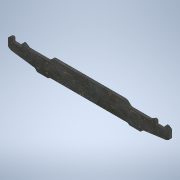
# Autodesk Inventor part: MK3 Rear Plate
Saved by Autodesk Inventor 2023 (Build 270158000, 158)
## iProperties
Created: 2019-05-27
Part Number: MK3 Rear Plate
Material: Steel
Document SubType Name: Modeling
Designer: Parker
Density: 7.85 g/cm^3
Appearance: Plate
Author: Parker
Revision Number: ANY
Autodesk Inventor part; units mm, degrees
ref_plane "YZ Plane" through (0, 0, 0) normal (1, 0, 0) x (0, 1, 0)
ref_plane "XZ Plane" through (0, 0, 0) normal (0, 1, 0) x (-1, 0, 0)
ref_plane "XY Plane" through (0, 0, 0) normal (0, 0, 1) x (1, 0, 0)
sketch "Sketch5" plane through (0, 0, 0) normal (0, 0, 1) x (1, 0, 0)
  line L0 (-212.5, -25) -> (212.5, -25)
  line L1 (212.5, -25) -> (212.5, 25)
  line L2 (212.5, 25) -> (-212.5, 25)
  line L3 (-212.5, 25) -> (-212.5, -25)
  line L4 (-212.5, -25) -> (212.5, 25) construction
  line L5 (212.5, -25) -> (-212.5, 25) construction
  point P0 (0, 0)
  dimension "d22" = 425
  dimension "d23" = 50
  constraints: 12 end point, 2 midpoint, 2 parallel, 1 horizontal, 1 perpendicular
  measures "d22" distance of L1.end L2.end
  measures "d23" distance of L2.end L0.start
extrude "Extrusion3" add sketch "Sketch5" along normal blind 6.35
sketch "Sketch6" plane through (0, 0, 0) normal (0, 0, -1) x (-1, 0, 0)
  circle A0 centre (74, 14.9487) radius 2.75
  circle A1 centre (85, 10.04) radius 2.75
  circle A2 centre (96, 14.9487) radius 2.75
  circle A3 centre (-74, 14.9487) radius 2.75
  circle A4 centre (-85, 10.04) radius 2.75
  circle A5 centre (-96, 14.9487) radius 2.75
  circle A6 centre (-19.65, 8.0332) radius 2.75
  circle A7 centre (2.35, 8.037) radius 2.75
  circle A8 centre (2.35, -13.963) radius 2.75
  circle A9 centre (-19.6575, -13.9668) radius 2.75
  point P0 (-19.6575, -16.9668)
  point P1 (-19.65, 5.0332)
  point P2 (2.35, 5.037)
  point P3 (2.35, -16.963)
  constraints: 10 centre point, 20 other
hole "Hole2" at (96, 14.9487, 0) at (85, 10.04, 0) at (74, 14.9487, 0) at (-74, 14.9487, 0) at (-85, 10.04, 0) at (-96, 14.9487, 0) at (-2.35, -13.963, 0) at (19.6575, -13.9668, 0) at (19.65, 8.0332, 0) at (-2.35, 8.037, 0) direction (0, 0, 1) diameter 3.2 end through all
sketch "Sketch7" plane through (0, 0, 0) normal (0, 0, -1) x (-1, 0, 0)
  circle A0 centre (-133.6, 8.1) radius 3.825
  circle A1 centre (-110.4, 8.1) radius 3.825
  circle A2 centre (-110.4, -15.1) radius 3.825
  circle A3 centre (-133.6, -15.1) radius 3.825
  circle A4 centre (133.6, -15.1) radius 3.825
  circle A5 centre (110.4, -15.1) radius 3.825
  circle A6 centre (110.4, 8.1) radius 3.825
  circle A7 centre (133.6, 8.1) radius 3.825
  point P0 (0, 0)
  constraints: 8 centre point, 16 other
hole "Hole3" at (133.6, 8.1, 0) at (133.6, -15.1, 0) at (110.4, -15.1, 0) at (110.4, 8.1, 0) at (-110.4, 8.1, 0) at (-133.6, 8.1, 0) at (-133.6, -15.1, 0) at (-110.4, -15.1, 0) direction (0, 0, 1) diameter 5.4 end through all
sketch "Sketch8" plane through (0, 0, 0) normal (0, 0, -1) x (-1, 0, 0)
  circle A0 centre (-208.5036, 13.3515) radius 1.7
  circle A1 centre (-208.5036, -3.1485) radius 1.7
  circle A2 centre (-167.5036, -3.1485) radius 1.7
  circle A3 centre (-167.5036, 13.3515) radius 1.7
  circle A4 centre (167.4964, 13.3515) radius 1.7
  circle A5 centre (167.4964, -3.1485) radius 1.7
  circle A6 centre (208.4964, -3.1485) radius 1.7
  circle A7 centre (208.4964, 13.3515) radius 1.7
  point P0 (0, 0)
  constraints: 8 centre point, 16 other
hole "Hole4" at (208.5036, 13.3515, 0) at (208.5036, -3.1485, 0) at (167.5036, -3.1485, 0) at (167.5036, 13.3515, 0) at (-167.4964, 13.3515, 0) at (-167.4964, -3.1485, 0) at (-208.4964, -3.1485, 0) at (-208.4964, 13.3515, 0) direction (0, 0, 1) diameter 2.2 end through all
sketch "Sketch9" plane through (0, 0, 0) normal (0, 0, -1) x (-1, 0, 0)
  arc A0 (-210.5036, 16.8156) -> (-210.5036, 9.8874) centre (-208.5036, 13.3515) ccw
  line L0 (-210.5036, 16.8156) -> (-205.1272, 20.2721)
  arc A1 (-204.9977, 20.3312) -> (-205.1272, 20.2721) centre (-204.8568, 19.8515) ccw
  arc A2 (-204.8568, 20.3515) -> (-204.9977, 20.3312) centre (-204.8568, 19.8515) ccw
  line L1 (-204.8568, 20.3515) -> (-202.0036, 20.3515)
  circle A3 centre (208.4964, -3.1485) radius 1.1 projected
  circle A4 centre (167.4964, 13.3515) radius 1.1 projected
  circle A5 centre (-167.5036, -3.1485) radius 1.1 projected
  circle A6 centre (-208.5036, 13.3515) radius 1.1 projected
  circle A7 centre (-208.5036, -3.1485) radius 1.1 projected
  circle A8 centre (-167.5036, 13.3515) radius 1.1 projected
  circle A9 centre (167.4964, -3.1485) radius 1.1 projected
  circle A10 centre (208.4964, 13.3515) radius 1.1 projected
  circle A11 centre (133.6, -15.1) radius 2.7 projected
  circle A12 centre (110.4, 8.1) radius 2.7 projected
  circle A13 centre (-110.4, -15.1) radius 2.7 projected
  circle A14 centre (-133.6, 8.1) radius 2.7 projected
  circle A15 centre (-133.6, -15.1) radius 2.7 projected
  circle A16 centre (-110.4, 8.1) radius 2.7 projected
  circle A17 centre (133.6, 8.1) radius 2.7 projected
  circle A18 centre (110.4, -15.1) radius 2.7 projected
  circle A19 centre (85, 10.04) radius 1.6 projected
  circle A20 centre (-74, 14.9487) radius 1.6 projected
  circle A21 centre (-96, 14.9487) radius 1.6 projected
  circle A22 centre (-85, 10.04) radius 1.6 projected
  circle A23 centre (74, 14.9487) radius 1.6 projected
  circle A24 centre (96, 14.9487) radius 1.6 projected
  line L2 (-212.5, -25) -> (-212.5, 25) projected
  line L3 (212.5, -25) -> (-212.5, -25) projected
  line L4 (212.5, 25) -> (212.5, -25) projected
  line L5 (-212.5, 25) -> (212.5, 25) projected
  line L6 (-174.0036, 20.3515) -> (-171.1505, 20.3515)
  arc A25 (-174.0036, 20.3515) -> (-174.448, 20.3015) centre (-174.0036, 18.3515) ccw
  arc A26 (-174.448, 20.3015) -> (-175.9536, 18.7959) centre (-174.0036, 18.3515) ccw
  arc A27 (-175.9536, 18.7959) -> (-176.0036, 18.3515) centre (-174.0036, 18.3515) ccw
  line L7 (-176.0036, 12.3515) -> (-176.0036, 18.3515)
  arc A28 (-201.5592, 20.3015) -> (-202.0036, 20.3515) centre (-202.0036, 18.3515) ccw
  arc A29 (-200.0536, 18.7959) -> (-201.5592, 20.3015) centre (-202.0036, 18.3515) ccw
  arc A30 (-200.0036, 18.3515) -> (-200.0536, 18.7959) centre (-202.0036, 18.3515) ccw
  line L8 (-200.0036, 18.3515) -> (-200.0036, 12.3515)
  line L9 (-198.0036, 10.3515) -> (-178.0036, 10.3515)
  circle A31 centre (-133.6, 8.1) radius 4.25
  circle A32 centre (-110.4, 8.1) radius 4.25
  line L10 (-161.2796, 14.1) -> (-106.2796, 14.1)
  line L11 (-106.2796, 14.1) -> (-95.3796, 25)
  arc A33 (-171.0096, 20.3312) -> (-171.1505, 20.3515) centre (-171.1505, 19.8515) ccw
  arc A34 (-170.8801, 20.2721) -> (-171.0096, 20.3312) centre (-171.1505, 19.8515) ccw
  line L12 (-170.8801, 20.2721) -> (-165.5036, 16.8156)
  line L13 (-165.5036, 16.8156) -> (-161.2796, 14.1)
  line L14 (-178.0036, 10.3515) -> (-178.0036, 10.3515)
  line L15 (-176.0036, 12.3515) -> (-176.0036, 12.3515)
  arc A35 (-178.0036, 10.3515) -> (-176.0036, 12.3515) centre (-178.0036, 12.3515) ccw
  line L16 (-198.0036, 10.3515) -> (-198.0036, 10.3515)
  line L17 (-200.0036, 12.3515) -> (-200.0036, 12.3515)
  arc A36 (-200.0036, 12.3515) -> (-198.0036, 10.3515) centre (-198.0036, 12.3515) ccw
  point P0 (0, 0)
  point P1 (-212.5, 13.5221)
  dimension "d47" = 6
  dimension "d48" = 45
  dimension "d49" = 2
  dimension "d50" = 2
  dimension "d51" = 55
  constraints: 29 end point, 26 point on circle, 15 centre point, 6 horizontal, 4 tangent, 2 perpendicular, 2 vertical, 1 collinear, 1 point on line, 49 other
  measures "d47" distance from line of L10 A31.centre
  measures "d48" angle of L5 L11
  measures "d49" radius of A35
  measures "d50" radius of A36
  measures "d51" distance of L10.start L10.end
extrude "Extrusion4" cut sketch "Sketch9" against normal through all contours A0 L2 L5 L11 L10 L13 L12 A34 A33 L6 A25 A26 A27 L7 A35 L9 A36 L8 A30 A29 A28 L1 A2 A1 L0
mirror "Mirror3" about plane through (0, 0, 0) normal (1, 0, 0) of "Extrusion4"
sketch "Sketch10" plane through (0, 0, 0) normal (0, 0, -1) x (-1, 0, 0)
  line L0 (212.5, -25) -> (-212.5, -25) projected
  line L1 (-136.6, -25) -> (-139.6, -19)
  line L2 (-139.6, -19) -> (-205.1276, -10.0894)
  line L3 (106.2796, 14.1) -> (95.3796, 25) projected
  line L4 (-95.3796, 25) -> (95.3796, 25) projected
  line L5 (-95.3796, 25) -> (-106.2796, 14.1) projected
  line L6 (-106.2796, 14.1) -> (-161.2796, 14.1) projected
  line L7 (-161.2796, 14.1) -> (-170.8801, 20.2721) projected
  arc A0 (-170.8801, 20.2721) -> (-171.1505, 20.3515) centre (-171.1505, 19.8515) ccw projected
  line L8 (-171.1505, 20.3515) -> (-174.0036, 20.3515) projected
  arc A1 (-174.0036, 20.3515) -> (-176.0036, 18.3515) centre (-174.0036, 18.3515) ccw projected
  line L9 (-176.0036, 18.3515) -> (-176.0036, 12.3515) projected
  arc A2 (-178.0036, 10.3515) -> (-176.0036, 12.3515) centre (-178.0036, 12.3515) ccw projected
  line L10 (-178.0036, 10.3515) -> (-198.0036, 10.3515) projected
  arc A3 (-200.0036, 12.3515) -> (-198.0036, 10.3515) centre (-198.0036, 12.3515) ccw projected
  line L11 (-200.0036, 12.3515) -> (-200.0036, 18.3515) projected
  arc A4 (-200.0036, 18.3515) -> (-202.0036, 20.3515) centre (-202.0036, 18.3515) ccw projected
  line L12 (-202.0036, 20.3515) -> (-204.8568, 20.3515) projected
  arc A5 (-204.8568, 20.3515) -> (-205.1272, 20.2721) centre (-204.8568, 19.8515) ccw projected
  line L13 (-205.1272, 20.2721) -> (-210.5036, 16.8156) projected
  arc A6 (-210.5036, 16.8156) -> (-212.5, 13.5221) centre (-208.5036, 13.3515) ccw projected
  line L14 (-212.5, -25) -> (-212.5, 13.5221) projected
  line L15 (212.5, -25) -> (-212.5, -25) projected
  line L16 (212.5, 13.5221) -> (212.5, -25) projected
  arc A7 (212.5, 13.5221) -> (210.5036, 16.8156) centre (208.5036, 13.3515) ccw projected
  line L17 (210.5036, 16.8156) -> (205.1272, 20.2721) projected
  arc A8 (205.1272, 20.2721) -> (204.8568, 20.3515) centre (204.8568, 19.8515) ccw projected
  line L18 (204.8568, 20.3515) -> (202.0036, 20.3515) projected
  arc A9 (202.0036, 20.3515) -> (200.0036, 18.3515) centre (202.0036, 18.3515) ccw projected
  line L19 (200.0036, 18.3515) -> (200.0036, 12.3515) projected
  arc A10 (198.0036, 10.3515) -> (200.0036, 12.3515) centre (198.0036, 12.3515) ccw projected
  line L20 (198.0036, 10.3515) -> (178.0036, 10.3515) projected
  arc A11 (176.0036, 12.3515) -> (178.0036, 10.3515) centre (178.0036, 12.3515) ccw projected
  line L21 (176.0036, 12.3515) -> (176.0036, 18.3515) projected
  arc A12 (176.0036, 18.3515) -> (174.0036, 20.3515) centre (174.0036, 18.3515) ccw projected
  line L22 (174.0036, 20.3515) -> (171.1505, 20.3515) projected
  arc A13 (171.1505, 20.3515) -> (170.8801, 20.2721) centre (171.1505, 19.8515) ccw projected
  line L23 (170.8801, 20.2721) -> (161.2796, 14.1) projected
  line L24 (161.2796, 14.1) -> (106.2796, 14.1) projected
  circle A14 centre (208.4964, -3.1485) radius 1.1 projected
  circle A15 centre (167.4964, 13.3515) radius 1.1 projected
  circle A16 centre (-167.5036, -3.1485) radius 1.1 projected
  circle A17 centre (-208.5036, 13.3515) radius 1.1 projected
  circle A18 centre (-208.5036, -3.1485) radius 1.1 projected
  circle A19 centre (-167.5036, 13.3515) radius 1.1 projected
  circle A20 centre (167.4964, -3.1485) radius 1.1 projected
  circle A21 centre (208.4964, 13.3515) radius 1.1 projected
  circle A22 centre (133.6, -15.1) radius 2.7 projected
  circle A23 centre (110.4, 8.1) radius 2.7 projected
  circle A24 centre (-110.4, -15.1) radius 2.7 projected
  circle A25 centre (-133.6, 8.1) radius 2.7 projected
  circle A26 centre (-133.6, -15.1) radius 2.7 projected
  circle A27 centre (-110.4, 8.1) radius 2.7 projected
  circle A28 centre (133.6, 8.1) radius 2.7 projected
  circle A29 centre (110.4, -15.1) radius 2.7 projected
  circle A30 centre (85, 10.04) radius 1.6 projected
  circle A31 centre (-74, 14.9487) radius 1.6 projected
  circle A32 centre (-96, 14.9487) radius 1.6 projected
  circle A33 centre (-85, 10.04) radius 1.6 projected
  circle A34 centre (74, 14.9487) radius 1.6 projected
  circle A35 centre (96, 14.9487) radius 1.6 projected
  arc A36 (-210.5036, 0.3156) -> (-210.5036, -6.6126) centre (-208.5036, -3.1485) ccw
  line L25 (-205.1276, -10.0894) -> (-210.5036, -6.6126)
  point P0 (0, 0)
  point P1 (-212.5, -3.3191)
  point P2 (-212.5, -25)
  dimension "d54" = 6
  dimension "d55" = 3
  dimension "d56" = 6
  constraints: 6 end point, 2 point on circle, 2 point on line, 1 centre point, 6 other
  measures "d54" horizontal distance of A26.centre L1.end
  measures "d55" horizontal distance of L1.end L1.start
  measures "d56" vertical distance of L1.start L1.end
extrude "Extrusion5" cut sketch "Sketch10" against normal blind 10 contours L0 L14 A36 L25 L2 L1
mirror "Mirror4" about plane through (0, 0, 0) normal (1, 0, 0) of "Extrusion5"
fillet "Fillet2" radius 10 2 edges at (205.1276, -10.0894, 3.175) (-205.1276, -10.0894, 3.175)
fillet "Fillet3" radius 10 2 edges at (-139.6, -19, 3.175) (139.6, -19, 3.175)
fillet "Fillet4" radius 10 6 edges at (106.2796, 14.1, 3.175) (95.3796, 25, 3.175) (-95.3796, 25, 3.175) (-106.2796, 14.1, 3.175) (-161.2796, 14.1, 3.175) (161.2796, 14.1, 3.175)
sketch "Sketch11" plane through (0, 0, 0) normal (0, 0, -1) x (-1, 0, 0)
  line L0 (136.6, -25) -> (-136.6, -25) projected
  line L1 (-106.9, -25) -> (-103.4, -21.5)
  line L2 (-103.4, -21.5) -> (103.4, -21.5)
  line L3 (103.4, -21.5) -> (106.9, -25)
  circle A0 centre (-110.4, -15.1) radius 2.7 projected
  circle A1 centre (110.4, -15.1) radius 2.7 projected
  point P0 (0, 0)
  dimension "d62" = 3.5
  dimension "d63" = 45
  dimension "d64" = 7
  dimension "d65" = 7
  constraints: 6 end point, 2 point on line, 1 parallel, 1 perpendicular
  measures "d62" distance between parallel lines of L0 L2
  measures "d63" angle of L0 L1
  measures "d64" horizontal distance of A0.centre L1.end
  measures "d65" horizontal distance of A1.centre L2.end
extrude "Extrusion6" cut sketch "Sketch11" against normal blind 10 contours L0 L1 L2 L3
fillet "Fillet5" radius 10 2 edges at (103.4, -21.5, 3.175) (-103.4, -21.5, 3.175)
sketch "Sketch12" plane through (0, 0, 0) normal (0, 0, -1) x (-1, 0, 0)
  circle A0 centre (110.4, -15.1) radius 2.7 projected
  line L0 (-99.2579, -21.5) -> (99.2579, -21.5) projected
  point P0 (0, 0)
  point P1 (80.4, -17.5)
  point P2 (80.4, -9.5)
  dimension "d69" = 8
  dimension "d70" = 30
  dimension "d71" = 4
  constraints: 1 vertical alignment
  measures "d69" distance of point (80.4, -9.5) point (80.4, -17.5)
  measures "d70" horizontal distance of A0.centre point (80.4, -17.5)
  measures "d71" distance from line of L0 point (80.4, -17.5)
hole "Hole5" at (-80.4, -17.5, 0) at (-80.4, -9.5, 0) direction (0, 0, 1) diameter 3.5 end through all
sketch "Sketch13" plane through (0, 0, 0) normal (0, 0, -1) x (-1, 0, 0)
  circle A0 centre (-7.9962, 0.635) radius 1.8
  circle A1 centre (-7.9962, 21) radius 1.8
  point P0 (0, 0)
  constraints: 2 centre point, 4 other
hole "Hole6" at (7.9962, 0.635, 0) at (7.9962, 21, 0) direction (0, 0, 1) diameter 1.8 end through all
body "Solid2"
